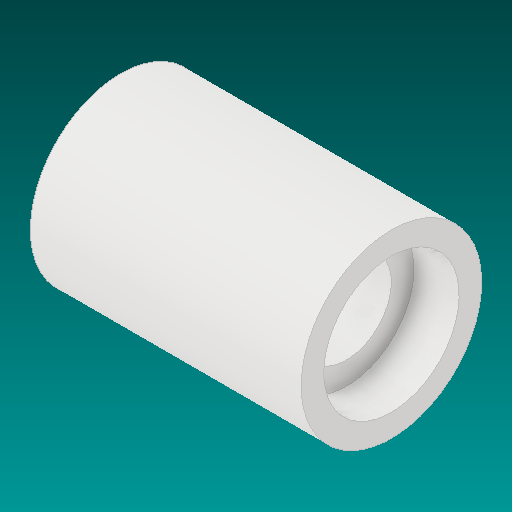
# Autodesk Inventor part: RORPOS20-L30_1
Saved by Autodesk Inventor 2020 (Build 240168000, 168)
## iProperties
Created: 2022-11-16
Part Number: RORPOS20-L30_1
Material: Generic
Catalog Web Link: www.cadenas.de
Description: RORPOS, RORPHS, RORPES, RORPJS, RORPSS, RORPQS, RORMCS_1-Plastic Roller -Milled/Straight-
Vendor: MISUMI
Document SubType Name: Modeling
Designer: psAdmin
Manufacturer: MISUMI
Mass: 6.08684 g
Surface Area: 34.5575 cm^2
Volume: 6.08684 cm^3
Density: 1 g/cm^3
Appearance: PSOLRGB-255-255-255
Category: PARTsolutions
Company: MISUMI
PSOL_IDENT_0: {$CADENAS_DATA/23d-libs/misumi/metric/53_rollers/rorpos.prj},227 {VTYP=3D},{NB=RORPOS20-L30_1},{LINA=
PSOL_IDENT_1: RORPOS20-L30},{NN=RORPOS, RORPHS, RORPES, RORPJS, RORPSS, RORPQS, RORMCS_1},{DATE=30.06.2021 13:26:5
PSOL_IDENT_2: 0},{GEOMDATE=18.05.2012 00:00:00},{VERSION=},{LINEID=10},{WBVAR=MAT,MATB,L},{WBNUMERIC=L}  {NB=RORPO
PSOL_IDENT_3: S20-L30_1},{LINA=RORPOS20-L30},{KT=DUMMY},{PN=RORPOS20-L30},{TYPE=RORPOS},{MAT=1},{ALT1=},{MATB=S},{
PSOL_IDENT_4: MATBALG= 'S', 'Steel', 'SS', 'Stainless Steel' },{NO=20},{NOM=20},{L=30},{L0=[15-100/1]},{BU=B696ZZx
PSOL_IDENT_5: 2},{BUN=696ZZ},{D=20},{D1=15},{DD=6},{B=5},{DDHH=10},{MATB1=Steel},{MATB2=52100 Bearing Steel}
NB: RORPOS20-L30_1
NN: RORPOS, RORPHS, RORPES, RORPJS, RORPSS, RORPQS, RORMCS_1
NT: Plastic Roller -Milled/Straight-
NBSYN: $PN._1
LINA: RORPOS20-L30
CATALOG: Misumi
PN: RORPOS20-L30
MAT: Polyacetal
MATB: Steel
NO: 20
L: 30
BU: B696ZZx2
D: 20
D1: 0
DD: 6
B: 5
DDHH: 10
SUPPLIER: MISUMI
ARTICLENO: RORPOS20-L30_1
BOMINFO: RORPOS20-L30
CREATOR: CADENAS GmbH
d2: 0.000 mm
Title: RORPOS20-L30
Author: Cadenas PARTsolutions
Comments: Plastic Roller -Milled/Straight-
Autodesk Inventor part; units mm, degrees
ref_plane "YZ Plane" through (0, 0, 0) normal (1, 0, 0) x (0, 1, 0)
ref_plane "XZ Plane" through (0, 0, 0) normal (0, 1, 0) x (-1, 0, 0)
ref_plane "XY Plane" through (0, 0, 0) normal (0, 0, 1) x (1, 0, 0)
sketch "Sketch_1" plane through (0, 0, 0) normal (0, 0, 1) x (1, 0, 0)
  line L0 (30, 0) -> (0, 0)
  line L1 (0, 7.5) -> (5, 7.5)
  line L2 (5, 7.5) -> (5, 5)
  line L3 (5, 5) -> (25, 5)
  line L4 (25, 5) -> (25, 7.5)
  line L5 (25, 7.5) -> (30, 7.5)
  line L6 (30, 7.5) -> (30, 10)
  line L7 (30, 10) -> (0, 10)
  line L8 (0, 10) -> (0, 7.5)
  constraints: 18 end point
revolve "Revolution1" add sketch "Sketch_1" angle 360 about axis through (30, 0, 0) along (1, 0, 0)
ref_plane "body_to_B_L__XY" through (0, 0, 0) normal (1, 0, 0) x (0, 0, -1)
ref_plane "body_to_B_L__YZ" through (0, 0, 0) normal (0, 0, -1) x (0, 1, 0)
ref_plane "body_to_B_L__ZX" through (0, 0, 0) normal (0, 1, 0) x (1, 0, 0)
ref_plane "body_to_B_R__XY" through (25, 0, 0) normal (-1, 0, 0) x (0, 0, -1)
ref_plane "body_to_B_R__YZ" through (25, 0, 0) normal (0, 0, -1) x (0, -1, 0)
ref_plane "body_to_B_R__ZX" through (25, 0, 0) normal (0, -1, 0) x (-1, 0, 0)
body "Solid1"
